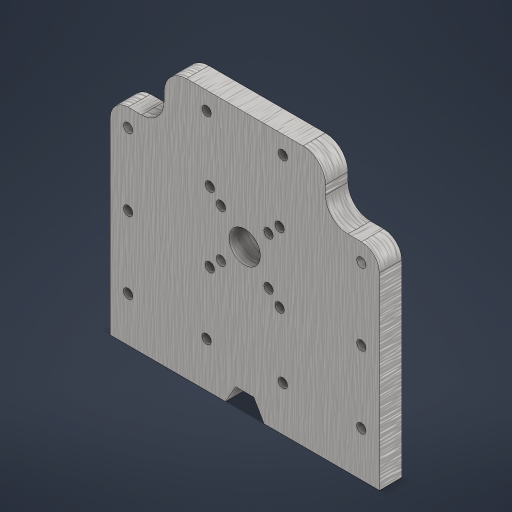
# Autodesk Inventor part: FirstStageMotorMountingPlate
Saved by Autodesk Inventor 2024 (Build 280153000, 153)
## iProperties
Created: 2024-01-05
Part Number: FirstStageMotorMountingPlate
Material: Aluminum 6061
Document SubType Name: Modeling
Designer: avsar
Density: 2.7 g/cm^3
Appearance: Satin Brushed
Author: avsar
Autodesk Inventor part; units mm, degrees
ref_plane "YZ Plane" through (0, 0, 0) normal (1, 0, 0) x (0, 1, 0)
ref_plane "XZ Plane" through (0, 0, 0) normal (0, 1, 0) x (-1, 0, 0)
ref_plane "XY Plane" through (0, 0, 0) normal (0, 0, 1) x (1, 0, 0)
sketch "Sketch1" plane through (0, 0, 0) normal (0, 0, 1) x (1, 0, 0)
  line L0 (-60, -46) -> (60, -46)
  line L1 (60, -46) -> (60, 46)
  line L2 (60, 46) -> (-60, 46)
  line L3 (-60, 46) -> (-60, -46)
  line L4 (-60, -46) -> (60, 46) construction
  line L5 (60, -46) -> (-60, 46) construction
  point P0 (0, 0)
  dimension "d0" = 120
  dimension "d1" = 92
  constraints: 12 end point, 2 midpoint, 2 parallel, 1 horizontal, 1 perpendicular
  measures "d0" distance of L2.end L1.end
  measures "d1" distance of L1.end L0.end
extrude "Extrusion1" add sketch "Sketch1" along normal mid plane 10
sketch "Sketch2" plane through (0, 0, 5) normal (0, 0, 1) x (1, 0, 0)
  circle A0 centre (0, 18) radius 7
  line L0 (-60, -46) -> (60, -46) projected
  circle A1 centre (-10.6066, 28.6066) radius 2.1
  line L1 (-10.6066, 28.6066) -> (0, 18) construction
  circle A2 centre (-15.5563, 33.5563) radius 2.1
  line L2 (-15.5563, 33.5563) -> (-10.6066, 28.6066) construction
  circle A3 centre (-15.5563, 2.4437) radius 2.1
  circle A4 centre (-10.6066, 7.3934) radius 2.1
  circle A5 centre (15.5563, 2.4437) radius 2.1
  circle A6 centre (10.6066, 7.3934) radius 2.1
  circle A7 centre (15.5563, 33.5563) radius 2.1
  circle A8 centre (10.6066, 28.6066) radius 2.1
  point P0 (0, 0)
  point P1 (0, -46)
  dimension "d4" = 14
  dimension "d6" = 64
  dimension "d7" = 4.2
  dimension "d8" = 45
  dimension "d9" = 15
  dimension "d10" = 4.2
  dimension "d11" = 7
  dimension "d14" = 360
  constraints: 9 centre point, 4 end point, 1 collinear, 1 midpoint, 1 vertical alignment, 17 other
  measures "d4" diameter of A0
  measures "d6" distance of point (0, -46) L1.end
  measures "d7" diameter of A1
  measures "d8" angle of L0 L1
  measures "d9" distance of L1.start L1.end
  measures "d10" diameter of A2
  measures "d11" distance of L2.start L1.start
extrude "Extrusion2" cut sketch "Sketch2" against normal through all
sketch "Sketch5" plane through (0, 0, 5) normal (0, 0, 1) x (1, 0, 0)
  line L0 (-60, -46) -> (60, -46) projected
  line L1 (-8.6188, -46) -> (-4, -38)
  line L2 (-4, -38) -> (4, -38)
  line L3 (4, -38) -> (8.6188, -46)
  point P0 (0, 0)
  point P1 (0, -38)
  point P2 (0, -46)
  dimension "d42" = 8
  dimension "d43" = 8
  dimension "d44" = 60
  constraints: 6 end point, 2 midpoint, 2 point on line, 1 equal length, 1 parallel, 1 vertical alignment
  measures "d42" distance between parallel lines of L0 L2
  measures "d43" distance of L1.end L2.end
  measures "d44" angle of L0 L3
extrude "Extrusion5" cut sketch "Sketch5" against normal through all
sketch "Sketch7" plane through (60, -46, -5) normal (0, -1, 0) x (1, 0, 0)
  circle A0 centre (-6, 5) radius 2
  line L0 (0, 0) -> (-51.3812, 0) construction
  circle A1 centre (-18, 5) radius 2
  circle A2 centre (-30, 5) radius 2
  circle A3 centre (-42, 5) radius 2
  circle A4 centre (-54, 5) radius 2 construction
  circle A5 centre (-66, 5) radius 2 construction
  circle A6 centre (-78, 5) radius 2
  circle A7 centre (-90, 5) radius 2
  circle A8 centre (-102, 5) radius 2
  circle A9 centre (-114, 5) radius 2
  line L1 (-54, 5) -> (-66, 5) construction
  point P0 (-60, 5)
  point P1 (-60, 5)
  dimension "d74" = 4
  dimension "d77" = 12
  constraints: 10 centre point, 2 end point, 2 horizontal, 1 coincident, 1 midpoint, 18 other
  measures "d74" diameter of A0
  measures "d77" distance of A0.centre A1.centre
extrude "Extrusion7" cut sketch "Sketch7" against normal blind 8
sketch "Sketch8" plane through (0, 0, 5) normal (0, 0, 1) x (1, 0, 0)
  circle A0 centre (-52, 38) radius 2.1
  line L0 (-60, 46) -> (-60, -46) construction
  line L1 (-60, -46) -> (-8.6188, -46) projected
  circle A1 centre (-52, 6) radius 2.1
  circle A2 centre (-52, -26) radius 2.1
  circle A3 centre (0, 18) radius 7 construction
  line L2 (0, 25) -> (0, 18) construction
  circle A4 centre (52, 38) radius 2.1
  circle A5 centre (52, 6) radius 2.1
  circle A6 centre (52, -26) radius 2.1
  point P0 (0, 0)
  dimension "d84" = 4.2
  dimension "d85" = 8
  dimension "d86" = 84
  dimension "d89" = 32
  constraints: 6 centre point, 3 symmetric about line, 2 end point, 2 vertical, 1 vertical alignment, 8 other
  measures "d84" diameter of A0
  measures "d85" distance from line of L0 A0.centre
  measures "d86" distance from line of L1 A0.centre
  measures "d89" distance of A0.centre A1.centre
extrude "Extrusion8" cut sketch "Sketch8" against normal through all
sketch "Sketch9" plane through (0, 0, 5) normal (0, 0, 1) x (1, 0, 0)
  line L0 (-36, 46) -> (36, 46)
  line L1 (36, 46) -> (36, 70)
  line L2 (36, 70) -> (-36, 70)
  line L3 (-36, 70) -> (-36, 46)
  line L4 (-36, 46) -> (36, 70) construction
  line L5 (36, 46) -> (-36, 70) construction
  line L6 (60, 46) -> (-60, 46) construction
  point P0 (0, 0)
  point P1 (0, 58)
  point P2 (0, 46)
  dimension "d96" = 72
  dimension "d97" = 24
  constraints: 12 end point, 4 midpoint, 2 parallel, 1 horizontal, 1 perpendicular, 1 vertical alignment
  measures "d96" distance of L2.end L1.end
  measures "d97" distance of L0.end L1.end
extrude "Extrusion9" add sketch "Sketch9" against normal up to surface (10 mm away)
sketch "Sketch10" plane through (0, 0, 5) normal (0, 0, 1) x (1, 0, 0)
  circle A0 centre (0, 18) radius 7 construction
  circle A1 centre (-17, 62) radius 2.1
  line L0 (-7, 18) -> (0, 18) construction
  line L1 (0, 18) -> (0, 25) construction
  circle A2 centre (17, 62) radius 2.1
  circle A3 centre (-17, -26) radius 2.1
  circle A4 centre (17, -26) radius 2.1
  point P0 (0, 0)
  dimension "d100" = 4.2
  dimension "d101" = 44
  dimension "d102" = 17
  constraints: 4 centre point, 4 end point, 3 symmetric about line, 2 point on circle, 1 horizontal, 1 perpendicular, 3 other
  measures "d100" diameter of A1
  measures "d101" vertical distance of A1.centre L0.end
  measures "d102" horizontal distance of L0.end A1.centre
extrude "Extrusion10" cut sketch "Sketch10" against normal blind 10
fillet "Fillet1" radius 10 4 edges at (36, 46, 0) (-36, 46, 0) (-36, 70, 0) (36, 70, 0)
fillet "Fillet2" radius 8 2 edges at (-60, 46, 0) (60, 46, 0)
thread "Thread9" size "M4.5x0.75" class "6H" standard "ISO Metric profile" full length
thread "Thread10" size "M4.5x0.75" class "6H" standard "ISO Metric profile" full length
body "Solid1"
